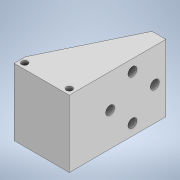
# Autodesk Inventor part: Finger_right_v5
Saved by Autodesk Inventor 2022 (Build 260153000, 153)
## iProperties
Created: 2022-06-04
Part Number: Finger_right_v5
Material: Generic
Document SubType Name: Modeling
Designer: kylem
Density: 1 g/cm^3
Appearance: Default
Author: kylem
Autodesk Inventor part; units mm, degrees
ref_plane "YZ Plane" through (0, 0, 0) normal (1, 0, 0) x (0, 1, 0)
ref_plane "XZ Plane" through (0, 0, 0) normal (0, 1, 0) x (-1, 0, 0)
sketch "Sketch1" plane through (0, 0, 0) normal (0, 1, 0) x (-1, 0, 0)
  line L0 (0, 0) -> (0, -30.6)
  line L1 (0, -30.6) -> (5, -30.6)
  line L2 (0, 0) -> (19.774, 0)
  line L3 (19.774, 0) -> (5, -30.6)
  line L4 (19.774, 0) -> (19.774, 4)
  line L5 (0, 0) -> (0, 9.5471)
  line L6 (19.774, 4) -> (-4.8744, 4)
  point P0 (0, 4)
  dimension "d0" = 30.6
  dimension "d1" = 5
  dimension "d2" = 19.774
  dimension "d3" = 4
  constraints: 14 end point, 2 horizontal, 2 perpendicular, 2 vertical
  measures "d0" distance of L0.start L0.end
  measures "d1" distance of L0.end L1.end
  measures "d2" distance of L0.start L2.end
  measures "d3" distance of L2.end L4.end
extrude "Extrusion1" add sketch "Sketch1" along normal blind 24
sketch "Sketch2" plane through (0, 0, 4) normal (1, 0, 0) x (0, 0, -1)
  line L0 (34.6, 0) -> (34.6, 24) projected
  line L1 (34.6, 12) -> (30.6, 12)
  line L2 (30.6, 12) -> (14.6, 12)
  line L3 (22.6, 12) -> (22.6, 20)
  line L4 (22.6, 12) -> (22.6, 4)
  circle A0 centre (22.6, 20) radius 1.6
  circle A1 centre (14.6, 12) radius 1.6
  circle A2 centre (22.6, 4) radius 1.6
  circle A3 centre (30.6, 12) radius 1.6
  point P0 (4, 0)
  dimension "d6" = 4
  dimension "d7" = 16
  dimension "d8" = 8
  dimension "d9" = 8
  dimension "d10" = 3.2
  dimension "d11" = 3.2
  dimension "d12" = 3.2
  dimension "d13" = 3.2
  constraints: 8 end point, 4 centre point, 4 coincident, 2 horizontal, 2 midpoint, 2 vertical
  measures "d6" distance of L1.start L1.end
  measures "d7" distance of L1.end L2.end
  measures "d8" distance of L3.start L3.end
  measures "d9" distance of L3.start L4.end
  measures "d10" diameter of A0
  measures "d11" diameter of A1
  measures "d12" diameter of A2
  measures "d13" diameter of A3
extrude "Extrusion2" cut sketch "Sketch2" against normal blind 24
ref_plane "Work Plane1" through (-3, 0, 4) normal (1, 0, 0) x (0, 0, -1)
sketch "Sketch3" plane through (-3, 0, 4) normal (1, 0, 0) x (0, 0, -1)
  circle A0 centre (22.6, 20) radius 1.6 projected
  circle A1 centre (22.6, 20) radius 2.95
  circle A2 centre (14.6, 12) radius 1.6 projected
  circle A3 centre (14.6, 12) radius 2.95
  circle A4 centre (22.6, 4) radius 1.6 projected
  circle A5 centre (22.6, 4) radius 2.95
  circle A6 centre (30.6, 12) radius 1.6 projected
  circle A7 centre (30.6, 12) radius 2.95
  point P0 (4, 0)
  dimension "d17" = 5.9
  dimension "d18" = 5.9
  dimension "d19" = 5.9
  dimension "d20" = 5.9
  constraints: 4 centre point, 4 coincident
  measures "d17" diameter of A1
  measures "d18" diameter of A3
  measures "d19" diameter of A5
  measures "d20" diameter of A7
extrude "Extrusion3" cut sketch "Sketch3" against normal blind 24 contours A0 | A1 | A2 | A3 | A4 | A5 | A6 | A7
sketch "Sketch4" plane through (0, 24, 0) normal (0, 1, 0) x (1, 0, 0)
  line L0 (0, -4) -> (0, 30.6) projected
  line L1 (0, -4) -> (-2, -4)
  line L2 (-2, -4) -> (-2, -2)
  line L3 (-2, -2) -> (0, -2)
  line L4 (0, -2) -> (0, -4)
  circle A0 centre (-2, -2) radius 1.1
  line L5 (-2, -2) -> (-18, -2)
  circle A1 centre (-18, -2) radius 1.1
  point P0 (0, 0)
  dimension "d23" = 2
  dimension "d24" = 2
  dimension "d25" = 2.2
  dimension "d26" = 16
  dimension "d27" = 2.2
  constraints: 10 end point, 2 centre point, 2 coincident, 2 horizontal, 2 parallel, 1 perpendicular
  measures "d23" distance of L2.end L3.end
  measures "d24" distance of L1.end L2.end
  measures "d25" diameter of A0
  measures "d26" distance of L5.start L5.end
  measures "d27" diameter of A1
extrude "Extrusion4" cut sketch "Sketch4" against normal blind 24 contours A1 | A0 L2 L3 | L3 L5 A0 | A0 L5 L2
body "Solid1"
